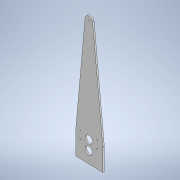
# Autodesk Inventor part: 関節3_側板2
Saved by Autodesk Inventor 2021 (Build 250183000, 183)
## iProperties
Created: 2022-01-31
Part Number: 関節3_側板2
Material: 一般
Document SubType Name: Modeling
Designer: hirohumi
Density: 1 g/cm^3
Appearance: 既定
Author: hirohumi
Autodesk Inventor part; units mm, degrees
ref_plane "YZ Plane" through (0, 0, 0) normal (1, 0, 0) x (0, 1, 0)
ref_plane "XZ Plane" through (0, 0, 0) normal (0, 1, 0) x (-1, 0, 0)
ref_plane "XY Plane" through (0, 0, 0) normal (0, 0, 1) x (1, 0, 0)
sketch "スケッチ1" plane through (0, 0, 0) normal (0, 0, 1) x (1, 0, 0)
  circle A0 centre (0, 0) radius 50 construction
  circle A1 centre (0, 25) radius 11.9375 construction
  circle A2 centre (0, 300) radius 5 construction
  circle A3 centre (0, 300) radius 47.7465 construction
  line L0 (47.4611, 294.7873) -> (11.8661, -29.3033) construction
  line L1 (-47.4611, 294.7873) -> (-11.8661, -29.3033) construction
  circle A4 centre (0, 25) radius 19.25 construction
  line L2 (-12.0776, 316.763) -> (11.6547, 316.763) construction
  line L3 (-22.6185, -92.0395) -> (22.1946, -92.0395) construction
  circle A5 centre (0, 300) radius 1.75
  arc A6 (37.1489, 26.0707) -> (37.1246, 26.5634) centre (32.1489, 26.0707) ccw
  arc A7 (-34.9787, 30.4606) -> (-35, 30) centre (-30, 30) ccw
  arc A8 (9.9513, 300.9854) -> (-9.9575, 300.9212) centre (0, 300) ccw
  line L4 (-9.9575, 300.9212) -> (-34.9787, 30.4606)
  line L5 (9.9513, 300.9854) -> (37.1246, 26.5634)
  line L6 (-35, 30) -> (-35, -30)
  line L7 (37.1489, -31.89) -> (37.1489, 26.0707)
  circle A9 centre (-9.1924, 34.1924) radius 1.6 construction
  circle A10 centre (9.1924, 34.1924) radius 1.6 construction
  line L8 (9.1924, 34.1924) -> (-9.1924, 34.1924) construction
  line L9 (-9.1924, 34.1924) -> (-9.1924, 15.8076) construction
  line L10 (-9.1924, 15.8076) -> (9.1924, 15.8076) construction
  line L11 (9.1924, 15.8076) -> (9.1924, 34.1924) construction
  line L12 (9.1924, 34.1924) -> (-9.1924, 15.8076) construction
  line L13 (-9.1924, 34.1924) -> (9.1924, 15.8076) construction
  circle A11 centre (0, 25) radius 13 construction
  circle A12 centre (-9.1924, 15.8076) radius 1.6 construction
  circle A13 centre (9.1924, 15.8076) radius 1.6 construction
  circle A14 centre (0, 25) radius 10.05
  circle A15 centre (0, 0) radius 4 construction
  circle A16 centre (0, 0) radius 10
  line L14 (22.5, 35) -> (-22.5, 35) construction
  line L15 (-22.5, 35) -> (-22.5, 15) construction
  line L16 (-22.5, 15) -> (22.5, 15) construction
  line L17 (22.5, 15) -> (22.5, 35) construction
  line L18 (22.5, 35) -> (-22.5, 15) construction
  line L19 (-22.5, 35) -> (22.5, 15) construction
  circle A17 centre (-22.5, 35) radius 1.6
  circle A18 centre (-22.5, 15) radius 1.6
  circle A19 centre (22.5, 35) radius 1.6
  circle A20 centre (22.5, 15) radius 1.6
  line L20 (-35, -30) -> (37.1489, -31.89)
  dimension "d38" = 26
  dimension "d1" = 100
  dimension "d3" = 23.875
  dimension "d8" = 10
  dimension "d9" = 300
  dimension "d10" = 95.493
  dimension "d11" = 38.5
  dimension "d25" = 3.5
  dimension "d26" = 5
  dimension "d28" = 10
  dimension "d29" = 5
  dimension "d35" = 25
  dimension "d36" = 3.2
  dimension "d37" = 3.2
  dimension "d39" = 3.2
  dimension "d40" = 3.2
  dimension "d41" = 20.1
  dimension "d42" = 8
  dimension "d43" = 20
  dimension "d44" = 45
  dimension "d45" = 20
  dimension "d46" = 3.2
  dimension "d47" = 3.2
  dimension "d48" = 3.2
  dimension "d49" = 3.2
  constraints: 42 end point, 20 centre point, 17 coincident, 8 point on circle, 7 tangent, 5 parallel, 4 horizontal, 4 midpoint, 3 perpendicular, 2 vertical alignment, 1 vertical, 3 other
  measures "d1" diameter of A0
  measures "d3" diameter of A1
  measures "d8" diameter of A2
  measures "d9" distance of point (0, 0) A2.centre
  measures "d10" diameter of A3
  measures "d11" diameter of A4
  measures "d25" diameter of A5
  measures "d26" radius of A6
  measures "d28" radius of A8
  measures "d29" radius of A7
  measures "d35" distance of point (0, 0) A1.centre
  measures "d36" diameter of A9
  measures "d37" diameter of A10
  measures "d39" diameter of A12
  measures "d40" diameter of A13
  measures "d41" diameter of A14
  measures "d42" diameter of A15
  measures "d43" diameter of A16
  measures "d44" distance of L16.end L15.end
  measures "d45" distance of L15.end L14.end
  measures "d46" diameter of A17
  measures "d47" diameter of A18
  measures "d48" diameter of A19
  measures "d49" diameter of A20
extrude "押し出し1" add sketch "スケッチ1" along normal blind 4
